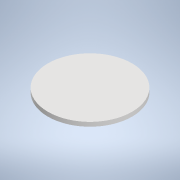
# Autodesk Inventor part: 5inCompliantWheelHub
Saved by Autodesk Inventor 2021 (Build 250183000, 183)
## iProperties
Created: 2020-09-12
Part Number: 5inCompliantWheelHub
Material: Generic
Document SubType Name: Modeling
Designer: deli
Density: 1 g/cm^3
Appearance: Default
Author: deli
Autodesk Inventor part; units mm, degrees
ref_plane "YZ Plane" through (0, 0, 0) normal (1, 0, 0) x (0, 1, 0)
ref_plane "XZ Plane" through (0, 0, 0) normal (0, 1, 0) x (-1, 0, 0)
ref_plane "XY Plane" through (0, 0, 0) normal (0, 0, 1) x (1, 0, 0)
sketch "Sketch1" plane through (0, 0, 0) normal (0, 1, 0) x (-1, 0, 0)
  circle A0 centre (-65.9389, 138.5386) radius 14 projected
  circle A1 centre (-65.9389, 138.5386) radius 13.746
  circle A2 centre (-65.9389, 138.5386) radius 31.75
  point P0 (0, 0)
  dimension "d0" = 27.492
  dimension "d1" = 28
  dimension "d2" = 63.5
  constraints: 2 centre point, 2 coincident
  measures "d0" diameter of A1
  measures "d1" diameter of A0
  measures "d2" diameter of A2
extrude "Extrusion1" add sketch "Sketch1" along normal blind 3.175 contours A0 | A1 | A2
sketch "Sketch2" plane through (65.9389, 0, 138.5386) normal (0, -1, 0) x (1, 0, 0)
  circle A0 centre (0, 0) radius 13.746
  point P0 (-65.9389, -138.5386)
  dimension "d5" = 27.492
  constraints: 1 centre point
  measures "d5" diameter of A0
extrude "Extrusion2" add sketch "Sketch2" along normal blind 38.1
sketch "Sketch3" plane through (65.9389, 0, 138.5386) normal (0, -1, 0) x (1, 0, 0)
  circle A0 centre (0, 23.8125) radius 2.1526 projected
  circle A1 centre (20.6222, 11.9062) radius 2.1526 projected
  circle A2 centre (20.6222, -11.9063) radius 2.1526 projected
  circle A3 centre (0, -23.8125) radius 2.1526 projected
  circle A4 centre (-20.6222, -11.9062) radius 2.1526 projected
  circle A5 centre (-20.6222, 11.9063) radius 2.1526 projected
  circle A6 centre (0, 23.8125) radius 1.8986
  circle A7 centre (20.6222, 11.9062) radius 1.8986
  circle A8 centre (20.6222, -11.9063) radius 1.8986
  circle A9 centre (-20.6222, -11.9062) radius 1.8986
  circle A10 centre (-20.6222, 11.9063) radius 1.8986
  circle A11 centre (0, -23.8125) radius 1.8986
  point P0 (-65.9389, -138.5386)
  dimension "d8" = 4.3053
  dimension "d9" = 3.7973
  dimension "d10" = 3.7973
  dimension "d11" = 3.7973
  dimension "d12" = 3.7973
  dimension "d13" = 3.7973
  dimension "d14" = 3.7973
  constraints: 6 centre point, 6 coincident
  measures "d8" diameter of A0
  measures "d9" diameter of A6
  measures "d10" diameter of A7
  measures "d11" diameter of A8
  measures "d12" diameter of A9
  measures "d13" diameter of A10
  measures "d14" diameter of A11
extrude "Extrusion3" add sketch "Sketch3" along normal blind 12.7 contours A6 | A7 | A8 | A9 | A10 | A11
body "Solid1"
